Autodesk Inventor part; units mm, degrees
(part 2 of 6)
sketch "Sketch18" plane through (0, 0, 19) normal (0, 0, 1) x (1, 0, 0)
  line L0 (103.6499, -134.3094) -> (100.1144, -130.7739) projected
  line L1 (100.1144, -130.7739) -> (91.3463, -139.542) projected
  line L2 (91.3463, -139.542) -> (94.8818, -143.0776) projected
  line L3 (94.8818, -143.0776) -> (103.6499, -134.3094) projected
  line L4 (96.296, -141.6633) -> (94.8818, -145.906) projected
  line L5 (94.8818, -145.906) -> (106.4783, -134.3094) projected
  line L6 (106.4783, -134.3094) -> (102.2357, -135.7236) projected
  line L7 (102.2357, -135.7236) -> (96.296, -141.6633) projected
  line L8 (101.5286, -129.3597) -> (100.1144, -130.7739) projected
  line L9 (100.1144, -130.7739) -> (102.2357, -132.8952) projected
  line L10 (102.2357, -132.8952) -> (106.4783, -134.3094) projected
  line L11 (106.4783, -134.3094) -> (101.5286, -129.3597) projected
  line L12 (106.4783, -134.3094) -> (102.2357, -135.7236) projected
  line L13 (102.2357, -132.8952) -> (106.4783, -134.3094) projected
  line L14 (102.2357, -135.7236) -> (102.2357, -132.8952) projected
  line L15 (89.9321, -140.9562) -> (91.3463, -139.542) projected
  line L16 (89.9321, -140.9562) -> (94.8818, -145.906) projected
  line L17 (94.8818, -145.906) -> (93.4676, -141.6633) projected
  line L18 (93.4676, -141.6633) -> (91.3463, -139.542) projected
  line L19 (94.8818, -145.906) -> (93.4676, -141.6633) projected
  line L20 (96.296, -141.6633) -> (94.8818, -145.906) projected
  line L21 (93.4676, -141.6633) -> (96.296, -141.6633) projected
  line L22 (6.2, -154.1002) -> (-6.2, -154.1002) projected
  line L23 (-6.2, -154.1002) -> (-6.2, -159.1002) projected
  line L24 (-6.2, -159.1002) -> (6.2, -159.1002) projected
  line L25 (6.2, -159.1002) -> (6.2, -154.1002) projected
  line L26 (-102.2357, -132.8952) -> (-102.2357, -135.7236) projected
  line L27 (-106.4783, -134.3094) -> (-102.2357, -132.8952) projected
  line L28 (-102.2357, -135.7236) -> (-106.4783, -134.3094) projected
  line L29 (-102.2357, -135.7236) -> (-106.4783, -134.3094) projected
  line L30 (-106.4783, -134.3094) -> (-94.8818, -145.906) projected
  line L31 (-94.8818, -145.906) -> (-96.296, -141.6633) projected
  line L32 (-96.296, -141.6633) -> (-102.2357, -135.7236) projected
  line L33 (-89.9321, -140.9562) -> (-91.3463, -139.542) projected
  line L34 (-91.3463, -139.542) -> (-93.4676, -141.6633) projected
  line L35 (-93.4676, -141.6633) -> (-94.8818, -145.906) projected
  line L36 (-94.8818, -145.906) -> (-89.9321, -140.9562) projected
  line L37 (-103.6499, -134.3094) -> (-94.8818, -143.0776) projected
  line L38 (-94.8818, -143.0776) -> (-91.3463, -139.542) projected
  line L39 (-91.3463, -139.542) -> (-100.1144, -130.7739) projected
  line L40 (-100.1144, -130.7739) -> (-103.6499, -134.3094) projected
  line L41 (-101.5286, -129.3597) -> (-100.1144, -130.7739) projected
  line L42 (-101.5286, -129.3597) -> (-106.4783, -134.3094) projected
  line L43 (-106.4783, -134.3094) -> (-102.2357, -132.8952) projected
  line L44 (-102.2357, -132.8952) -> (-100.1144, -130.7739) projected
  line L45 (-89.9321, -1.6439) -> (-91.3463, -3.0581) projected
  line L46 (-89.9321, -1.6439) -> (-94.8818, 3.3058) projected
  line L47 (-94.8818, 3.3058) -> (-93.4676, -0.9368) projected
  line L48 (-93.4676, -0.9368) -> (-91.3463, -3.0581) projected
  line L49 (-96.296, -0.9368) -> (-94.8818, 3.3058) projected
  line L50 (-94.8818, 3.3058) -> (-106.4783, -8.2907) projected
  line L51 (-106.4783, -8.2907) -> (-102.2357, -6.8765) projected
  line L52 (-102.2357, -6.8765) -> (-96.296, -0.9368) projected
  line L53 (-101.5286, -13.2405) -> (-100.1144, -11.8263) projected
  line L54 (-100.1144, -11.8263) -> (-102.2357, -9.7049) projected
  line L55 (-102.2357, -9.7049) -> (-106.4783, -8.2907) projected
  line L56 (-106.4783, -8.2907) -> (-101.5286, -13.2405) projected
  line L57 (-103.6499, -8.2907) -> (-100.1144, -11.8263) projected
  line L58 (-100.1144, -11.8263) -> (-91.3463, -3.0581) projected
  line L59 (-91.3463, -3.0581) -> (-94.8818, 0.4774) projected
  line L60 (-94.8818, 0.4774) -> (-103.6499, -8.2907) projected
  line L61 (91.3463, -3.0581) -> (100.1144, -11.8263) projected
  line L62 (100.1144, -11.8263) -> (103.6499, -8.2907) projected
  line L63 (103.6499, -8.2907) -> (94.8818, 0.4774) projected
  line L64 (94.8818, 0.4774) -> (91.3463, -3.0581) projected
  line L65 (-6.2, 11.5) -> (6.2, 11.5) projected
  line L66 (6.2, 11.5) -> (6.2, 16.5) projected
  line L67 (6.2, 16.5) -> (-6.2, 16.5) projected
  line L68 (-6.2, 16.5) -> (-6.2, 11.5) projected
  point P0 (0, 0)
  point P1 (-106.4783, -8.2907)
extrude "Extrusion17" cut sketch "Sketch18" against normal blind 9
sketch "Sketch27" plane through (0, 0, 19) normal (0, 0, 1) x (1, 0, 0)
  arc A0 (0.7519, -14.6599) -> (-0.7481, -14.6599) centre (0.0019, -13.9985) ccw
  arc A1 (-0.7481, 14.663) -> (0.7519, 14.663) centre (0.0019, 14.0015) ccw
  arc A2 (-76.7327, -25.4047) -> (-77.7933, -26.4653) centre (-77.7307, -25.4673) ccw
  arc A3 (-77.723, -116.1493) -> (-76.6623, -117.21) centre (-77.6603, -117.1473) ccw
  arc A4 (-0.7284, -128.0101) -> (0.7716, -128.0101) centre (0.0216, -128.6716) ccw
  arc A5 (76.7885, -117.2378) -> (77.8491, -116.1771) centre (77.7865, -117.1752) ccw
  arc A6 (77.8163, -26.5003) -> (76.7557, -25.4397) centre (77.7537, -25.5023) ccw
  arc A7 (97.4901, -4.7053) -> (98.5507, -5.7659) centre (97.5527, -5.7033) ccw
  arc A8 (-98.5277, -5.7309) -> (-97.4671, -4.6703) centre (-97.5297, -5.6683) ccw
  arc A9 (-97.3967, -137.9444) -> (-98.4574, -136.8837) centre (-97.4593, -136.9463) ccw
  arc A10 (0.7716, -157.333) -> (-0.7284, -157.333) centre (0.0216, -156.6716) ccw
  arc A11 (98.5835, -136.9115) -> (97.5229, -137.9722) centre (97.5855, -136.9741) ccw
  point P0 (0, 0)
  constraints: 24 point on circle, 12 centre point, 48 other
hole "Hole4" at (0.0216, -128.6716, 19) at (77.7865, -117.1752, 19) at (77.7537, -25.5023, 19) at (0.0019, -13.9985, 19) at (-77.7307, -25.4673, 19) at (-77.6603, -117.1473, 19) direction (0, 0, -1) diameter 3 depth 24
sketch "Sketch28" plane through (0, 0, -5) normal (0, 0, -1) x (-1, 0, 0)
  circle A0 centre (-0.0019, -13.9985) radius 1.5 projected
  circle A1 centre (77.7307, -25.4673) radius 1.5 projected
  circle A2 centre (77.6603, -117.1473) radius 1.5 projected
  circle A3 centre (-0.0216, -128.6716) radius 1.5 projected
  circle A4 centre (-77.7865, -117.1752) radius 1.5 projected
  circle A5 centre (-77.7537, -25.5023) radius 1.5 projected
  line L0 (3.2486, -14.0007) -> (1.6214, -16.8146)
  line L1 (1.6214, -16.8146) -> (-1.6291, -16.8124)
  line L2 (-1.6291, -16.8124) -> (-3.2524, -13.9963)
  line L3 (-3.2524, -13.9963) -> (-1.6252, -11.1823)
  line L4 (-1.6252, -11.1823) -> (1.6252, -11.1846)
  line L5 (1.6252, -11.1846) -> (3.2486, -14.0007)
  line L6 (80.4442, -22.8741) -> (81.3332, -26.5207)
  line L7 (81.3332, -26.5207) -> (78.6197, -29.1139)
  line L8 (78.6197, -29.1139) -> (75.0172, -28.0605)
  line L9 (75.0172, -28.0605) -> (74.1282, -24.4139)
  line L10 (74.1282, -24.4139) -> (76.8417, -21.8207)
  line L11 (76.8417, -21.8207) -> (80.4442, -22.8741)
  line L12 (80.3739, -119.7405) -> (76.7714, -120.7939)
  line L13 (76.7714, -120.7939) -> (74.0578, -118.2007)
  line L14 (74.0578, -118.2007) -> (74.9468, -114.5542)
  line L15 (74.9468, -114.5542) -> (78.5493, -113.5008)
  line L16 (78.5493, -113.5008) -> (81.2629, -116.094)
  line L17 (81.2629, -116.094) -> (80.3739, -119.7405)
  line L18 (-0.0216, -132.2511) -> (-3.1216, -130.4614)
  line L19 (-3.1216, -130.4614) -> (-3.1216, -126.8818)
  line L20 (-3.1216, -126.8818) -> (-0.0216, -125.092)
  line L21 (-0.0216, -125.092) -> (3.0784, -126.8818)
  line L22 (3.0784, -126.8818) -> (3.0784, -130.4614)
  line L23 (3.0784, -130.4614) -> (-0.0216, -132.2511)
  line L24 (-78.6286, -113.5175) -> (-75.0399, -114.6171)
  line L25 (-75.0399, -114.6171) -> (-74.1979, -118.2748)
  line L26 (-74.1979, -118.2748) -> (-76.9445, -120.8328)
  line L27 (-76.9445, -120.8328) -> (-80.5331, -119.7332)
  line L28 (-80.5331, -119.7332) -> (-81.3752, -116.0755)
  line L29 (-81.3752, -116.0755) -> (-78.6286, -113.5175)
  line L30 (-76.9117, -21.8446) -> (-74.165, -24.4027)
  line L31 (-74.165, -24.4027) -> (-75.0071, -28.0604)
  line L32 (-75.0071, -28.0604) -> (-78.5957, -29.16)
  line L33 (-78.5957, -29.16) -> (-81.3424, -26.6019)
  line L34 (-81.3424, -26.6019) -> (-80.5003, -22.9442)
  line L35 (-80.5003, -22.9442) -> (-76.9117, -21.8446)
  circle A6 centre (77.7307, -25.4673) radius 1.5 projected
  circle A7 centre (-77.7537, -25.5023) radius 1.5 projected
  circle A8 centre (-0.0216, -128.6716) radius 1.5 projected
  circle A9 centre (-77.7865, -117.1752) radius 1.5 projected
  circle A10 centre (-0.0019, -13.9985) radius 1.5 projected
  circle A11 centre (77.6603, -117.1473) radius 1.5 projected
  circle A12 centre (0, 5.5) radius 5 projected
  circle A13 centre (-91.4877, -130.9153) radius 5 projected
  circle A14 centre (91.4877, -130.9153) radius 5 projected
  circle A15 centre (91.4877, -11.6848) radius 5 projected
  circle A16 centre (0, -148.1002) radius 5 projected
  circle A17 centre (-91.4877, -11.6848) radius 5 projected
  line L36 (-90.7904, -117.2044) -> (-78.2393, -130.6805)
  line L37 (-90.7904, -25.3958) -> (-78.2393, -11.9196)
  line L38 (90.9578, -25.2283) -> (78.2393, -11.9196)
  line L39 (78.2393, -130.6805) -> (90.9578, -117.3718)
  line L40 (-9.202, -138.2888) -> (9.202, -138.2888)
  point P0 (0, 0)
  point P1 (0, -11.1835)
  dimension "d396" = 3.2505
  dimension "d397" = 3.2505
  dimension "d398" = 3.2505
  dimension "d400" = 3.2505
  dimension "d401" = 3.2505
  dimension "d416" = 3.1
  constraints: 82 end point, 6 coincident, 5 perpendicular, 1 horizontal, 1 midpoint, 1 vertical alignment, 78 other
  measures "d396" distance of L0.start A0.centre
  measures "d397" distance from line of L6 A1.centre
  measures "d398" distance from line of L17 A2.centre
  measures "d400" distance from line of A4.centre L26
  measures "d401" distance from line of L33 A5.centre
  measures "d416" distance from line of L21 A3.centre
extrude "Extrusion27" cut sketch "Sketch28" against normal blind 2.4 contours A0 | A1 | A2 | A3 | A4 | A5 | L0 L1 L2 L3 L4 L5 | L6 L7 L8 L9 L10 L11 | L12 L13 L14 L15 L16 L17 | L18 L19 L20 L21 L22 L23 | L24 L25 L26 L27 L28 L29 | L30 L31 L32 L33 L34 L35
sketch "Sketch30" plane through (0, 0, 10) normal (0, 0, 1) x (1, 0, 0)
  line L0 (-100.1144, -130.7739) -> (-83.8509, -114.5104) projected
  line L1 (-83.8509, -114.5104) -> (-80.3154, -110.9749) projected
  line L2 (-80.3154, -110.9749) -> (-71.5473, -119.743) projected
  line L3 (-71.5473, -119.743) -> (-75.0828, -123.2786) projected
  line L4 (-75.0828, -123.2786) -> (-91.3463, -139.542) projected
  line L5 (-100.1144, -130.7739) -> (-91.3463, -139.542) projected
  line L6 (-6.2, -154.1002) -> (-6.2, -131.1002) projected
  line L7 (-6.2, -131.1002) -> (-6.2, -126.1002) projected
  line L8 (-6.2, -126.1002) -> (6.2, -126.1002) projected
  line L9 (6.2, -126.1002) -> (6.2, -131.1002) projected
  line L10 (6.2, -131.1002) -> (6.2, -154.1002) projected
  line L11 (-6.2, -154.1002) -> (6.2, -154.1002) projected
  line L12 (-91.3463, -3.0581) -> (-75.0828, -19.3216) projected
  line L13 (-75.0828, -19.3216) -> (-71.5473, -22.8571) projected
  line L14 (-71.5473, -22.8571) -> (-80.3154, -31.6252) projected
  line L15 (-80.3154, -31.6252) -> (-83.8509, -28.0897) projected
  line L16 (-83.8509, -28.0897) -> (-100.1144, -11.8263) projected
  line L17 (-91.3463, -3.0581) -> (-100.1144, -11.8263) projected
  line L18 (91.3463, -139.542) -> (75.0828, -123.2786) projected
  line L19 (75.0828, -123.2786) -> (71.5473, -119.743) projected
  line L20 (71.5473, -119.743) -> (80.3154, -110.9749) projected
  line L21 (80.3154, -110.9749) -> (83.8509, -114.5104) projected
  line L22 (83.8509, -114.5104) -> (100.1144, -130.7739) projected
  line L23 (91.3463, -139.542) -> (100.1144, -130.7739) projected
  line L24 (76.8724, -48.8001) -> (88.2822, -48.8001) projected
  line L25 (88.2822, -48.8001) -> (94.3529, -27.4901) projected
  line L26 (94.3529, -27.4901) -> (106.8333, -15.0097) projected
  arc A0 (106.8333, -15.0097) -> (88.1629, 3.6608) centre (97.4981, -5.6744) ccw projected
  line L27 (88.1629, 3.6608) -> (75.6824, -8.8196) projected
  line L28 (75.6824, -8.8196) -> (57.202, -21.3001) projected
  line L29 (57.202, -21.3001) -> (38.202, -31.3001) projected
  line L30 (38.202, -31.3001) -> (19.202, -21.3001) projected
  line L31 (19.202, -21.3001) -> (13.202, -3.65) projected
  line L32 (13.202, -3.65) -> (13.202, 14) projected
  arc A1 (13.202, 14) -> (-13.202, 14) centre (0, 14) ccw projected
  line L33 (-13.202, 14) -> (-13.202, -3.65) projected
  line L34 (-13.202, -3.65) -> (-19.202, -21.3001) projected
  line L35 (-19.202, -21.3001) -> (-38.202, -31.3001) projected
  line L36 (-38.202, -31.3001) -> (-57.202, -21.3001) projected
  line L37 (-57.202, -21.3001) -> (-75.6824, -8.8196) projected
  line L38 (-75.6824, -8.8196) -> (-88.1629, 3.6608) projected
  arc A2 (-88.1629, 3.6608) -> (-106.8333, -15.0097) centre (-97.4981, -5.6744) ccw projected
  line L39 (-106.8333, -15.0097) -> (-94.3529, -27.4901) projected
  line L40 (-94.3529, -27.4901) -> (-76.3482, -71.3001) projected
  line L41 (-76.3482, -71.3001) -> (-94.3529, -115.1101) projected
  line L42 (-94.3529, -115.1101) -> (-106.8333, -127.5905) projected
  arc A3 (-106.8333, -127.5905) -> (-88.1629, -146.2609) centre (-97.4981, -136.9257) ccw projected
  line L43 (-88.1629, -146.2609) -> (-75.6824, -133.7805) projected
  line L44 (-75.6824, -133.7805) -> (-57.202, -121.3001) projected
  line L45 (-57.202, -121.3001) -> (-38.202, -111.3001) projected
  line L46 (-38.202, -111.3001) -> (-19.202, -121.3001) projected
  line L47 (-19.202, -121.3001) -> (-13.202, -138.9501) projected
  line L48 (-13.202, -138.9501) -> (-13.202, -156.6002) projected
  arc A4 (-13.202, -156.6002) -> (13.202, -156.6002) centre (0, -156.6002) ccw projected
  line L49 (13.202, -156.6002) -> (13.202, -138.9501) projected
  line L50 (13.202, -138.9501) -> (19.202, -121.3001) projected
  line L51 (19.202, -121.3001) -> (38.202, -111.3001) projected
  line L52 (38.202, -111.3001) -> (57.202, -121.3001) projected
  line L53 (57.202, -121.3001) -> (75.6824, -133.7805) projected
  line L54 (75.6824, -133.7805) -> (88.1629, -146.2609) projected
  arc A5 (88.1629, -146.2609) -> (106.8333, -127.5905) centre (97.4981, -136.9257) ccw projected
  line L55 (106.8333, -127.5905) -> (94.3529, -115.1101) projected
  line L56 (94.3529, -115.1101) -> (88.2822, -93.8001) projected
  line L57 (88.2822, -93.8001) -> (76.8724, -93.8001) projected
  line L58 (76.8724, -93.8001) -> (76.8724, -48.8001) projected
  line L59 (6.2, -16.5) -> (-6.2, -16.5) projected
  line L60 (-6.2, -16.5) -> (-6.2, -11.5) projected
  line L61 (-6.2, -11.5) -> (-6.2, 11.5) projected
  line L62 (6.2, 11.5) -> (-6.2, 11.5) projected
  line L63 (6.2, 11.5) -> (6.2, -11.5) projected
  line L64 (6.2, -11.5) -> (6.2, -16.5) projected
  line L65 (100.1144, -11.8263) -> (83.8509, -28.0897) projected
  line L66 (83.8509, -28.0897) -> (80.3154, -31.6252) projected
  line L67 (80.3154, -31.6252) -> (71.5473, -22.8571) projected
  line L68 (71.5473, -22.8571) -> (75.0828, -19.3216) projected
  line L69 (75.0828, -19.3216) -> (91.3463, -3.0581) projected
  line L70 (100.1144, -11.8263) -> (91.3463, -3.0581) projected
  line L71 (-6.2, 11.5) -> (6.2, 11.5)
  line L72 (6.2, 11.5) -> (6.2, 17.5)
  line L73 (6.2, 17.5) -> (-6.2, 17.5)
  line L74 (-6.2, 17.5) -> (-6.2, 11.5)
  line L75 (0, 11.5) -> (0, 17.5)
  line L76 (0, 17.5) -> (4.5, 17.5)
  line L77 (4.5, 17.5) -> (4.5, 11.5)
  line L78 (4.5, 11.5) -> (0, 11.5)
  line L79 (0, 11.5) -> (-4.5, 11.5)
  line L80 (-4.5, 11.5) -> (-4.5, 17.5)
  line L81 (-4.5, 17.5) -> (0, 17.5)
  line L82 (0, 17.5) -> (0, 11.5)
  line L83 (-100.1144, -11.8263) -> (-91.3463, -3.0581)
  line L84 (-91.3463, -3.0581) -> (-95.5889, 1.1845)
  line L85 (-95.5889, 1.1845) -> (-104.357, -7.5836)
  line L86 (-104.357, -7.5836) -> (-100.1144, -11.8263)
  line L87 (-95.7303, -7.4422) -> (-92.5483, -4.2602)
  line L88 (-92.5483, -4.2602) -> (-96.791, -0.0176)
  line L89 (-96.791, -0.0176) -> (-99.973, -3.1996)
  line L90 (-99.973, -3.1996) -> (-95.7303, -7.4422)
  line L91 (-95.7303, -7.4422) -> (-98.9123, -10.6242)
  line L92 (-98.9123, -10.6242) -> (-103.1549, -6.3815)
  line L93 (-103.1549, -6.3815) -> (-99.973, -3.1996)
  line L94 (-99.973, -3.1996) -> (-95.7303, -7.4422)
  line L95 (-100.1144, -130.7739) -> (-91.3463, -139.542)
  line L96 (-91.3463, -139.542) -> (-95.5889, -143.7847)
  line L97 (-95.5889, -143.7847) -> (-104.357, -135.0165)
  line L98 (-104.357, -135.0165) -> (-100.1144, -130.7739)
  line L99 (-95.7303, -135.158) -> (-98.9123, -131.976)
  line L100 (-98.9123, -131.976) -> (-103.1549, -136.2186)
  line L101 (-103.1549, -136.2186) -> (-99.973, -139.4006)
  line L102 (-99.973, -139.4006) -> (-95.7303, -135.158)
  line L103 (-95.7303, -135.158) -> (-99.973, -139.4006)
  line L104 (-99.973, -139.4006) -> (-96.791, -142.5826)
  line L105 (-96.791, -142.5826) -> (-92.5483, -138.3399)
  line L106 (-92.5483, -138.3399) -> (-95.7303, -135.158)
  line L107 (-6.2, -154.1002) -> (6.2, -154.1002)
  line L108 (6.2, -154.1002) -> (6.2, -160.1002)
  line L109 (6.2, -160.1002) -> (-6.2, -160.1002)
  line L110 (-6.2, -160.1002) -> (-6.2, -154.1002)
  line L111 (0, -154.1002) -> (0, -160.1002)
  line L112 (0, -160.1002) -> (-4.5, -160.1002)
  line L113 (-4.5, -160.1002) -> (-4.5, -154.1002)
  line L114 (-4.5, -154.1002) -> (0, -154.1002)
  line L115 (0, -154.1002) -> (0, -160.1002)
  line L116 (0, -160.1002) -> (4.5, -160.1002)
  line L117 (4.5, -160.1002) -> (4.5, -154.1002)
  line L118 (4.5, -154.1002) -> (0, -154.1002)
  line L119 (91.3463, -139.542) -> (100.1144, -130.7739)
  line L120 (100.1144, -130.7739) -> (104.357, -135.0165)
  line L121 (104.357, -135.0165) -> (95.5889, -143.7847)
  line L122 (95.5889, -143.7847) -> (91.3463, -139.542)
  line L123 (95.7303, -135.158) -> (99.973, -139.4006)
  line L124 (99.973, -139.4006) -> (96.791, -142.5826)
  line L125 (96.791, -142.5826) -> (92.5483, -138.3399)
  line L126 (92.5483, -138.3399) -> (95.7303, -135.158)
  line L127 (95.7303, -135.158) -> (99.973, -139.4006)
  line L128 (99.973, -139.4006) -> (103.1549, -136.2186)
  line L129 (103.1549, -136.2186) -> (98.9123, -131.976)
  line L130 (98.9123, -131.976) -> (95.7303, -135.158)
  line L131 (91.3463, -3.0581) -> (100.1144, -11.8263)
  line L132 (100.1144, -11.8263) -> (104.357, -7.5836)
  line L133 (104.357, -7.5836) -> (95.5889, 1.1845)
  line L134 (95.5889, 1.1845) -> (91.3463, -3.0581)
  line L135 (95.7303, -7.4422) -> (99.973, -3.1996)
  line L136 (99.973, -3.1996) -> (96.791, -0.0176)
  line L137 (96.791, -0.0176) -> (92.5483, -4.2602)
  line L138 (92.5483, -4.2602) -> (95.7303, -7.4422)
  line L139 (95.7303, -7.4422) -> (98.9123, -10.6242)
  line L140 (98.9123, -10.6242) -> (103.1549, -6.3815)
  line L141 (103.1549, -6.3815) -> (99.973, -3.1996)
  line L142 (99.973, -3.1996) -> (95.7303, -7.4422)
  point P0 (0, 0)
  point P1 (96.791, -0.0176)
  point P2 (-96.791, -142.5826)
  point P3 (-103.1549, -136.2186)
  point P4 (-96.791, -0.0176)
  point P5 (-103.1549, -6.3815)
  point P6 (4.5, 17.5)
  dimension "d455" = 6
  dimension "d456" = 4.5
  dimension "d457" = 4.5
  dimension "d458" = 1.7
  dimension "d459" = 12.4
  dimension "d460" = 6
  dimension "d461" = 4.5
  dimension "d462" = 4.5
  dimension "d463" = 6
  dimension "d464" = 4.5
  dimension "d465" = 4.5
  dimension "d466" = 6
  dimension "d467" = 4.5
  dimension "d468" = 4.5
  dimension "d472" = 6
  dimension "d473" = 4.5
  dimension "d474" = 4.5
  dimension "d475" = 4.5
  dimension "d476" = 4.5
  dimension "d477" = 6
  dimension "d478" = 154.5851
  dimension "d479" = 147.5831
  dimension "d480" = 147.5831
  constraints: 144 end point, 39 equal length, 24 perpendicular, 10 midpoint, 7 point on line
  measures "d455" distance of L72.end L62.start
  measures "d456" distance of L75.end L76.end
  measures "d457" distance of L75.start L79.end
  measures "d458" distance between parallel lines of L80 L74
  measures "d459" distance of L72.end L73.end
  measures "d460" distance of L84.end L12.start
  measures "d461" distance between parallel lines of L88 L90
  measures "d462" distance between parallel lines of L90 L92
  measures "d463" distance of L4.end L96.end
  measures "d464" distance between parallel lines of L100 L102
  measures "d465" distance between parallel lines of L102 L105
  measures "d466" distance of L10.end L108.end
  measures "d467" distance between parallel lines of L113 L111
  measures "d468" distance between parallel lines of L111 L117
  measures "d472" distance of L18.start L121.end
  measures "d473" distance between parallel lines of L125 L123
  measures "d474" distance between parallel lines of L129 L123
  measures "d475" distance between parallel lines of L137 L135
  measures "d476" distance between parallel lines of L135 L140
  measures "d477" distance of L133.end L69.end
  measures "d478" distance between parallel lines of L55 L101
  measures "d479" distance between parallel lines of L65 L89
  measures "d480" distance between parallel lines of L65 L93
extrude "Extrusion29" add sketch "Sketch30" along normal blind 9 contours L5 L100 L97 L98 | L5 L96 L97 L105 | L11 L113 L109 L110 | L11 L108 L109 L117 | L17 L88 L85 L84 | L17 L86 L85 L92 | L23 L125 L121 L122 | L23 L120 L121 L129 | L62 L77 L73 L72 | L74 L73 L80 L62 | L70 L140 L133 L132 | L70 L134 L133 L137
sketch "Sketch31" plane through (0, 0, 10) normal (0, 0, 1) x (1, 0, 0)
  line L0 (76.8724, -48.8001) -> (88.2822, -48.8001) projected
  line L1 (88.2822, -48.8001) -> (94.3529, -27.4901) projected
  line L2 (94.3529, -27.4901) -> (106.8333, -15.0097) projected
  arc A0 (106.8333, -15.0097) -> (88.1629, 3.6608) centre (97.4981, -5.6744) ccw projected
  line L3 (88.1629, 3.6608) -> (75.6824, -8.8196) projected
  line L4 (75.6824, -8.8196) -> (57.202, -21.3001) projected
  line L5 (57.202, -21.3001) -> (38.202, -31.3001) projected
  line L6 (38.202, -31.3001) -> (19.202, -21.3001) projected
  line L7 (19.202, -21.3001) -> (13.202, -3.65) projected
  line L8 (13.202, -3.65) -> (13.202, 14) projected
  arc A1 (13.202, 14) -> (-13.202, 14) centre (0, 14) ccw projected
  line L9 (-13.202, 14) -> (-13.202, -3.65) projected
  line L10 (-13.202, -3.65) -> (-19.202, -21.3001) projected
  line L11 (-19.202, -21.3001) -> (-38.202, -31.3001) projected
  line L12 (-38.202, -31.3001) -> (-57.202, -21.3001) projected
  line L13 (-57.202, -21.3001) -> (-75.6824, -8.8196) projected
  line L14 (-75.6824, -8.8196) -> (-88.1629, 3.6608) projected
  arc A2 (-88.1629, 3.6608) -> (-106.8333, -15.0097) centre (-97.4981, -5.6744) ccw projected
  line L15 (-106.8333, -15.0097) -> (-94.3529, -27.4901) projected
  line L16 (-94.3529, -27.4901) -> (-76.3482, -71.3001) projected
  line L17 (-76.3482, -71.3001) -> (-94.3529, -115.1101) projected
  line L18 (-94.3529, -115.1101) -> (-106.8333, -127.5905) projected
  arc A3 (-106.8333, -127.5905) -> (-88.1629, -146.2609) centre (-97.4981, -136.9257) ccw projected
  line L19 (-88.1629, -146.2609) -> (-75.6824, -133.7805) projected
  line L20 (-75.6824, -133.7805) -> (-57.202, -121.3001) projected
  line L21 (-57.202, -121.3001) -> (-38.202, -111.3001) projected
  line L22 (-38.202, -111.3001) -> (-19.202, -121.3001) projected
  line L23 (-19.202, -121.3001) -> (-13.202, -138.9501) projected
  line L24 (-13.202, -138.9501) -> (-13.202, -156.6002) projected
  arc A4 (-13.202, -156.6002) -> (13.202, -156.6002) centre (0, -156.6002) ccw projected
  line L25 (13.202, -156.6002) -> (13.202, -138.9501) projected
  line L26 (13.202, -138.9501) -> (19.202, -121.3001) projected
  line L27 (19.202, -121.3001) -> (38.202, -111.3001) projected
  line L28 (38.202, -111.3001) -> (57.202, -121.3001) projected
  line L29 (57.202, -121.3001) -> (75.6824, -133.7805) projected
  line L30 (75.6824, -133.7805) -> (88.1629, -146.2609) projected
  arc A5 (88.1629, -146.2609) -> (106.8333, -127.5905) centre (97.4981, -136.9257) ccw projected
  line L31 (106.8333, -127.5905) -> (94.3529, -115.1101) projected
  line L32 (94.3529, -115.1101) -> (88.2822, -93.8001) projected
  line L33 (88.2822, -93.8001) -> (76.8724, -93.8001) projected
  line L34 (76.8724, -93.8001) -> (76.8724, -48.8001) projected
  line L35 (-91.3463, -139.542) -> (-95.5889, -143.7847) projected
  line L36 (-95.5889, -143.7847) -> (-96.791, -142.5826) projected
  line L37 (-96.791, -142.5826) -> (-92.5483, -138.3399) projected
  line L38 (-98.9123, -131.976) -> (-92.5483, -138.3399) projected
  line L39 (-98.9123, -131.976) -> (-103.1549, -136.2186) projected
  line L40 (-103.1549, -136.2186) -> (-104.357, -135.0165) projected
  line L41 (-104.357, -135.0165) -> (-100.1144, -130.7739) projected
  line L42 (-100.1144, -130.7739) -> (-83.8509, -114.5104) projected
  line L43 (-83.8509, -114.5104) -> (-80.3154, -110.9749) projected
  line L44 (-80.3154, -110.9749) -> (-71.5473, -119.743) projected
  line L45 (-71.5473, -119.743) -> (-75.0828, -123.2786) projected
  line L46 (-75.0828, -123.2786) -> (-91.3463, -139.542) projected
  line L47 (100.1144, -130.7739) -> (104.357, -135.0165) projected
  line L48 (104.357, -135.0165) -> (103.1549, -136.2186) projected
  line L49 (103.1549, -136.2186) -> (98.9123, -131.976) projected
  line L50 (92.5483, -138.3399) -> (98.9123, -131.976) projected
  line L51 (92.5483, -138.3399) -> (96.791, -142.5826) projected
  line L52 (96.791, -142.5826) -> (95.5889, -143.7847) projected
  line L53 (95.5889, -143.7847) -> (91.3463, -139.542) projected
  line L54 (91.3463, -139.542) -> (75.0828, -123.2786) projected
  line L55 (75.0828, -123.2786) -> (71.5473, -119.743) projected
  line L56 (71.5473, -119.743) -> (80.3154, -110.9749) projected
  line L57 (80.3154, -110.9749) -> (83.8509, -114.5104) projected
  line L58 (83.8509, -114.5104) -> (100.1144, -130.7739) projected
  line L59 (-100.1144, -11.8263) -> (-104.357, -7.5836) projected
  line L60 (-104.357, -7.5836) -> (-103.1549, -6.3815) projected
  line L61 (-103.1549, -6.3815) -> (-98.9123, -10.6242) projected
  line L62 (-92.5483, -4.2602) -> (-98.9123, -10.6242) projected
  line L63 (-92.5483, -4.2602) -> (-96.791, -0.0176) projected
  line L64 (-96.791, -0.0176) -> (-95.5889, 1.1845) projected
  line L65 (-95.5889, 1.1845) -> (-91.3463, -3.0581) projected
  line L66 (-91.3463, -3.0581) -> (-75.0828, -19.3216) projected
  line L67 (-75.0828, -19.3216) -> (-71.5473, -22.8571) projected
  line L68 (-71.5473, -22.8571) -> (-80.3154, -31.6252) projected
  line L69 (-80.3154, -31.6252) -> (-83.8509, -28.0897) projected
  line L70 (-83.8509, -28.0897) -> (-100.1144, -11.8263) projected
  line L71 (6.2, 17.5) -> (6.2, 11.5) projected
  line L72 (6.2, 11.5) -> (6.2, -11.5) projected
  line L73 (6.2, -11.5) -> (6.2, -16.5) projected
  line L74 (6.2, -16.5) -> (-6.2, -16.5) projected
  line L75 (-6.2, -16.5) -> (-6.2, -11.5) projected
  line L76 (-6.2, -11.5) -> (-6.2, 11.5) projected
  line L77 (-6.2, 11.5) -> (-6.2, 17.5) projected
  line L78 (-6.2, 17.5) -> (-4.5, 17.5) projected
  line L79 (-4.5, 17.5) -> (-4.5, 11.5) projected
  line L80 (4.5, 11.5) -> (-4.5, 11.5) projected
  line L81 (4.5, 11.5) -> (4.5, 17.5) projected
  line L82 (4.5, 17.5) -> (6.2, 17.5) projected
  line L83 (104.357, -7.5836) -> (100.1144, -11.8263) projected
  line L84 (100.1144, -11.8263) -> (83.8509, -28.0897) projected
  line L85 (83.8509, -28.0897) -> (80.3154, -31.6252) projected
  line L86 (80.3154, -31.6252) -> (71.5473, -22.8571) projected
  line L87 (71.5473, -22.8571) -> (75.0828, -19.3216) projected
  line L88 (75.0828, -19.3216) -> (91.3463, -3.0581) projected
  line L89 (91.3463, -3.0581) -> (95.5889, 1.1845) projected
  line L90 (95.5889, 1.1845) -> (96.791, -0.0176) projected
  line L91 (96.791, -0.0176) -> (92.5483, -4.2602) projected
  line L92 (98.9123, -10.6242) -> (92.5483, -4.2602) projected
  line L93 (98.9123, -10.6242) -> (103.1549, -6.3815) projected
  line L94 (103.1549, -6.3815) -> (104.357, -7.5836) projected
  line L95 (-6.2, -160.1002) -> (-6.2, -154.1002) projected
  line L96 (-6.2, -154.1002) -> (-6.2, -131.1002) projected
  line L97 (-6.2, -131.1002) -> (-6.2, -126.1002) projected
  line L98 (-6.2, -126.1002) -> (6.2, -126.1002) projected
  line L99 (6.2, -126.1002) -> (6.2, -131.1002) projected
  line L100 (6.2, -131.1002) -> (6.2, -154.1002) projected
  line L101 (6.2, -154.1002) -> (6.2, -160.1002) projected
  line L102 (6.2, -160.1002) -> (4.5, -160.1002) projected
  line L103 (4.5, -160.1002) -> (4.5, -154.1002) projected
  line L104 (-4.5, -154.1002) -> (4.5, -154.1002) projected
  line L105 (-4.5, -154.1002) -> (-4.5, -160.1002) projected
  line L106 (-4.5, -160.1002) -> (-6.2, -160.1002) projected
  line L107 (-4.5, 11.5) -> (-4.5, 17.5)
  line L108 (-4.5, 17.5) -> (4.5, 17.5)
  line L109 (4.5, 17.5) -> (4.5, 11.5)
  line L110 (4.5, 11.5) -> (-4.5, 11.5)
  line L111 (-98.9123, -10.6242) -> (-92.5483, -4.2602)
  line L112 (-92.5483, -4.2602) -> (-96.791, -0.0176)
  line L113 (-96.791, -0.0176) -> (-103.1549, -6.3815)
  line L114 (-103.1549, -6.3815) -> (-98.9123, -10.6242)
  line L115 (-98.9123, -131.976) -> (-92.5483, -138.3399)
  line L116 (-92.5483, -138.3399) -> (-96.791, -142.5826)
  line L117 (-96.791, -142.5826) -> (-103.1549, -136.2186)
  line L118 (-103.1549, -136.2186) -> (-98.9123, -131.976)
  line L119 (-4.5, -154.1002) -> (4.5, -154.1002)
  line L120 (4.5, -154.1002) -> (4.5, -160.1002)
  line L121 (4.5, -160.1002) -> (-4.5, -160.1002)
  line L122 (-4.5, -160.1002) -> (-4.5, -154.1002)
  line L123 (92.5483, -138.3399) -> (98.9123, -131.976)
  line L124 (98.9123, -131.976) -> (103.1549, -136.2186)
  line L125 (103.1549, -136.2186) -> (96.791, -142.5826)
  line L126 (96.791, -142.5826) -> (92.5483, -138.3399)
  line L127 (98.9123, -10.6242) -> (103.1549, -6.3815)
  line L128 (103.1549, -6.3815) -> (96.791, -0.0176)
  line L129 (96.791, -0.0176) -> (92.5483, -4.2602)
  line L130 (92.5483, -4.2602) -> (98.9123, -10.6242)
  point P0 (0, 0)
  dimension "d483" = 154.5851
  dimension "d484" = 90.1087
  dimension "d485" = 10.7
  dimension "d486" = 147.5831
  dimension "d487" = 66.3001
  dimension "d488" = 72.3725
  constraints: 48 end point, 15 equal length, 9 perpendicular
  measures "d483" distance between parallel lines of L31 L117
  measures "d484" distance between parallel lines of L83 L125
  measures "d485" distance between parallel lines of L83 L129
  measures "d486" distance between parallel lines of L83 L113
  measures "d487" distance between parallel lines of L33 L121
  measures "d488" distance between parallel lines of L34 L109
extrude "Extrusion30" cut sketch "Sketch31" against normal blind 10 contours L117 L39 L38 L37 | L125 L51 L50 L49 | L113 L63 L62 L61 | L81 L80 L79 L108 | L93 L92 L91 L128 | L105 L104 L103 L121
sketch "Sketch32" plane through (0, 0, 19) normal (0, 0, 1) x (1, 0, 0)
  line L0 (4.5, 17.5) -> (4.5, 11.5) projected
  line L1 (4.5, 11.5) -> (6.2, 11.5) projected
  line L2 (6.2, 11.5) -> (6.2, 17.5) projected
  line L3 (6.2, 17.5) -> (4.5, 17.5) projected
  line L4 (-4.5, 17.5) -> (-6.2, 17.5) projected
  line L5 (-6.2, 17.5) -> (-6.2, 11.5) projected
  line L6 (-6.2, 11.5) -> (-4.5, 11.5) projected
  line L7 (-4.5, 11.5) -> (-4.5, 17.5) projected
  line L8 (-103.1549, -6.3815) -> (-104.357, -7.5836) projected
  line L9 (-104.357, -7.5836) -> (-100.1144, -11.8263) projected
  line L10 (-100.1144, -11.8263) -> (-98.9123, -10.6242) projected
  line L11 (-98.9123, -10.6242) -> (-103.1549, -6.3815) projected
  line L12 (-96.791, -0.0176) -> (-92.5483, -4.2602) projected
  line L13 (-92.5483, -4.2602) -> (-91.3463, -3.0581) projected
  line L14 (-91.3463, -3.0581) -> (-95.5889, 1.1845) projected
  line L15 (-95.5889, 1.1845) -> (-96.791, -0.0176) projected
  line L16 (-92.5483, -138.3399) -> (-96.791, -142.5826) projected
  line L17 (-96.791, -142.5826) -> (-95.5889, -143.7847) projected
  line L18 (-95.5889, -143.7847) -> (-91.3463, -139.542) projected
  line L19 (-91.3463, -139.542) -> (-92.5483, -138.3399) projected
  line L20 (-98.9123, -131.976) -> (-100.1144, -130.7739) projected
  line L21 (-100.1144, -130.7739) -> (-104.357, -135.0165) projected
  line L22 (-104.357, -135.0165) -> (-103.1549, -136.2186) projected
  line L23 (-103.1549, -136.2186) -> (-98.9123, -131.976) projected
  line L24 (-4.5, -154.1002) -> (-6.2, -154.1002) projected
  line L25 (-6.2, -154.1002) -> (-6.2, -160.1002) projected
  line L26 (-6.2, -160.1002) -> (-4.5, -160.1002) projected
  line L27 (-4.5, -160.1002) -> (-4.5, -154.1002) projected
  line L28 (4.5, -154.1002) -> (4.5, -160.1002) projected
  line L29 (4.5, -160.1002) -> (6.2, -160.1002) projected
  line L30 (6.2, -160.1002) -> (6.2, -154.1002) projected
  line L31 (6.2, -154.1002) -> (4.5, -154.1002) projected
  line L32 (92.5483, -138.3399) -> (91.3463, -139.542) projected
  line L33 (91.3463, -139.542) -> (95.5889, -143.7847) projected
  line L34 (95.5889, -143.7847) -> (96.791, -142.5826) projected
  line L35 (96.791, -142.5826) -> (92.5483, -138.3399) projected
  line L36 (98.9123, -131.976) -> (103.1549, -136.2186) projected
  line L37 (103.1549, -136.2186) -> (104.357, -135.0165) projected
  line L38 (104.357, -135.0165) -> (100.1144, -130.7739) projected
  line L39 (100.1144, -130.7739) -> (98.9123, -131.976) projected
  line L40 (98.9123, -10.6242) -> (100.1144, -11.8263) projected
  line L41 (100.1144, -11.8263) -> (104.357, -7.5836) projected
  line L42 (104.357, -7.5836) -> (103.1549, -6.3815) projected
  line L43 (103.1549, -6.3815) -> (98.9123, -10.6242) projected
  line L44 (92.5483, -4.2602) -> (96.791, -0.0176) projected
  line L45 (96.791, -0.0176) -> (95.5889, 1.1845) projected
  line L46 (95.5889, 1.1845) -> (91.3463, -3.0581) projected
  line L47 (91.3463, -3.0581) -> (92.5483, -4.2602) projected
  line L48 (-4.5, 17.5) -> (-4.5, 11.5)
  line L49 (-4.5, 11.5) -> (4.5, 11.5)
  line L50 (4.5, 11.5) -> (4.5, 17.5)
  line L51 (4.5, 17.5) -> (-4.5, 17.5)
  line L52 (-96.791, -0.0176) -> (-103.1549, -6.3815)
  line L53 (-103.1549, -6.3815) -> (-98.9123, -10.6242)
  line L54 (-98.9123, -10.6242) -> (-92.5483, -4.2602)
  line L55 (-92.5483, -4.2602) -> (-96.791, -0.0176)
  line L56 (-103.1549, -136.2186) -> (-96.791, -142.5826)
  line L57 (-96.791, -142.5826) -> (-92.5483, -138.3399)
  line L58 (-92.5483, -138.3399) -> (-98.9123, -131.976)
  line L59 (-98.9123, -131.976) -> (-103.1549, -136.2186)
  line L60 (-4.5, -160.1002) -> (4.5, -160.1002)
  line L61 (4.5, -160.1002) -> (4.5, -154.1002)
  line L62 (4.5, -154.1002) -> (-4.5, -154.1002)
  line L63 (-4.5, -154.1002) -> (-4.5, -160.1002)
  line L64 (98.9123, -131.976) -> (92.5483, -138.3399)
  line L65 (92.5483, -138.3399) -> (96.791, -142.5826)
  line L66 (96.791, -142.5826) -> (103.1549, -136.2186)
  line L67 (103.1549, -136.2186) -> (98.9123, -131.976)
  line L68 (92.5483, -4.2602) -> (98.9123, -10.6242)
  line L69 (98.9123, -10.6242) -> (103.1549, -6.3815)
  line L70 (103.1549, -6.3815) -> (96.791, -0.0176)
  line L71 (96.791, -0.0176) -> (92.5483, -4.2602)
  point P0 (0, 0)
  point P1 (96.791, -0.0176)
  dimension "d491" = 0
  dimension "d492" = 231.6918
  dimension "d493" = 91.8087
  dimension "d494" = 139.8831
  dimension "d495" = 171.6002
  dimension "d496" = 1.7
  constraints: 48 end point, 13 parallel, 10 perpendicular, 1 vertical
  measures "d491" distance between parallel lines of L42 L70
  measures "d492" distance between parallel lines of L42 L58
  measures "d493" distance between parallel lines of L43 L66
  measures "d494" distance between parallel lines of L43 L54
  measures "d495" distance between parallel lines of L3 L62
  measures "d496" distance between parallel lines of L2 L50
extrude "Extrusion31" add sketch "Sketch32" against normal blind 5 contours L0 L49 L7 L51 | L52 L12 L54 L11 | L16 L56 L23 L58 | L62 L28 L60 L27 | L64 L36 L66 L35 | L68 L44 L70 L43
sketch "Sketch35" plane through (0, 0, 10) normal (0, 0, 1) x (1, 0, 0)
  line L0 (-103.1549, -6.3815) -> (-96.791, -0.0176) projected
  line L1 (-96.791, -0.0176) -> (-95.5889, 1.1845) projected
  line L2 (-95.5889, 1.1845) -> (-91.3463, -3.0581) projected
  line L3 (-91.3463, -3.0581) -> (-75.0828, -19.3216) projected
  line L4 (-75.0828, -19.3216) -> (-71.5473, -22.8571) projected
  line L5 (-71.5473, -22.8571) -> (-80.3154, -31.6252) projected
  line L6 (-80.3154, -31.6252) -> (-83.8509, -28.0897) projected
  line L7 (-83.8509, -28.0897) -> (-100.1144, -11.8263) projected
  line L8 (-100.1144, -11.8263) -> (-104.357, -7.5836) projected
  line L9 (-104.357, -7.5836) -> (-103.1549, -6.3815) projected
  line L10 (4.5, -160.1002) -> (-4.5, -160.1002) projected
  line L11 (-4.5, -160.1002) -> (-6.2, -160.1002) projected
  line L12 (-6.2, -160.1002) -> (-6.2, -154.1002) projected
  line L13 (-6.2, -154.1002) -> (-6.2, -131.1002) projected
  line L14 (-6.2, -131.1002) -> (-6.2, -126.1002) projected
  line L15 (-6.2, -126.1002) -> (6.2, -126.1002) projected
  line L16 (6.2, -126.1002) -> (6.2, -131.1002) projected
  line L17 (6.2, -131.1002) -> (6.2, -154.1002) projected
  line L18 (6.2, -154.1002) -> (6.2, -160.1002) projected
  line L19 (6.2, -160.1002) -> (4.5, -160.1002) projected
  line L20 (96.791, -0.0176) -> (103.1549, -6.3815) projected
  line L21 (103.1549, -6.3815) -> (104.357, -7.5836) projected
  line L22 (104.357, -7.5836) -> (100.1144, -11.8263) projected
  line L23 (100.1144, -11.8263) -> (83.8509, -28.0897) projected
  line L24 (83.8509, -28.0897) -> (80.3154, -31.6252) projected
  line L25 (80.3154, -31.6252) -> (71.5473, -22.8571) projected
  line L26 (71.5473, -22.8571) -> (75.0828, -19.3216) projected
  line L27 (75.0828, -19.3216) -> (91.3463, -3.0581) projected
  line L28 (91.3463, -3.0581) -> (95.5889, 1.1845) projected
  line L29 (95.5889, 1.1845) -> (96.791, -0.0176) projected
  line L30 (76.8724, -48.8001) -> (88.2822, -48.8001) projected
  line L31 (88.2822, -48.8001) -> (94.3529, -27.4901) projected
  line L32 (94.3529, -27.4901) -> (106.8333, -15.0097) projected
  arc A0 (106.8333, -15.0097) -> (88.1629, 3.6608) centre (97.4981, -5.6744) ccw projected
  line L33 (88.1629, 3.6608) -> (75.6824, -8.8196) projected
  line L34 (75.6824, -8.8196) -> (57.202, -21.3001) projected
  line L35 (57.202, -21.3001) -> (38.202, -31.3001) projected
  line L36 (38.202, -31.3001) -> (19.202, -21.3001) projected
  line L37 (19.202, -21.3001) -> (13.202, -3.65) projected
  line L38 (13.202, -3.65) -> (13.202, 14) projected
  arc A1 (13.202, 14) -> (-13.202, 14) centre (0, 14) ccw projected
  line L39 (-13.202, 14) -> (-13.202, -3.65) projected
  line L40 (-13.202, -3.65) -> (-19.202, -21.3001) projected
  line L41 (-19.202, -21.3001) -> (-38.202, -31.3001) projected
  line L42 (-38.202, -31.3001) -> (-57.202, -21.3001) projected
  line L43 (-57.202, -21.3001) -> (-75.6824, -8.8196) projected
  line L44 (-75.6824, -8.8196) -> (-88.1629, 3.6608) projected
  arc A2 (-88.1629, 3.6608) -> (-106.8333, -15.0097) centre (-97.4981, -5.6744) ccw projected
  line L45 (-106.8333, -15.0097) -> (-94.3529, -27.4901) projected
  line L46 (-94.3529, -27.4901) -> (-76.3482, -71.3001) projected
  line L47 (-76.3482, -71.3001) -> (-94.3529, -115.1101) projected
  line L48 (-94.3529, -115.1101) -> (-106.8333, -127.5905) projected
  arc A3 (-106.8333, -127.5905) -> (-88.1629, -146.2609) centre (-97.4981, -136.9257) ccw projected
  line L49 (-88.1629, -146.2609) -> (-75.6824, -133.7805) projected
  line L50 (-75.6824, -133.7805) -> (-57.202, -121.3001) projected
  line L51 (-57.202, -121.3001) -> (-38.202, -111.3001) projected
  line L52 (-38.202, -111.3001) -> (-19.202, -121.3001) projected
  line L53 (-19.202, -121.3001) -> (-13.202, -138.9501) projected
  line L54 (-13.202, -138.9501) -> (-13.202, -156.6002) projected
  arc A4 (-13.202, -156.6002) -> (13.202, -156.6002) centre (0, -156.6002) ccw projected
  line L55 (13.202, -156.6002) -> (13.202, -138.9501) projected
  line L56 (13.202, -138.9501) -> (19.202, -121.3001) projected
  line L57 (19.202, -121.3001) -> (38.202, -111.3001) projected
  line L58 (38.202, -111.3001) -> (57.202, -121.3001) projected
  line L59 (57.202, -121.3001) -> (75.6824, -133.7805) projected
  line L60 (75.6824, -133.7805) -> (88.1629, -146.2609) projected
  arc A5 (88.1629, -146.2609) -> (106.8333, -127.5905) centre (97.4981, -136.9257) ccw projected
  line L61 (106.8333, -127.5905) -> (94.3529, -115.1101) projected
  line L62 (94.3529, -115.1101) -> (88.2822, -93.8001) projected
  line L63 (88.2822, -93.8001) -> (76.8724, -93.8001) projected
  line L64 (76.8724, -93.8001) -> (76.8724, -48.8001) projected
  line L65 (-96.791, -142.5826) -> (-103.1549, -136.2186) projected
  line L66 (-103.1549, -136.2186) -> (-104.357, -135.0165) projected
  line L67 (-104.357, -135.0165) -> (-100.1144, -130.7739) projected
  line L68 (-100.1144, -130.7739) -> (-83.8509, -114.5104) projected
  line L69 (-83.8509, -114.5104) -> (-80.3154, -110.9749) projected
  line L70 (-80.3154, -110.9749) -> (-71.5473, -119.743) projected
  line L71 (-71.5473, -119.743) -> (-75.0828, -123.2786) projected
  line L72 (-75.0828, -123.2786) -> (-91.3463, -139.542) projected
  line L73 (-91.3463, -139.542) -> (-95.5889, -143.7847) projected
  line L74 (-95.5889, -143.7847) -> (-96.791, -142.5826) projected
  line L75 (103.1549, -136.2186) -> (96.791, -142.5826) projected
  line L76 (96.791, -142.5826) -> (95.5889, -143.7847) projected
  line L77 (95.5889, -143.7847) -> (91.3463, -139.542) projected
  line L78 (91.3463, -139.542) -> (75.0828, -123.2786) projected
  line L79 (75.0828, -123.2786) -> (71.5473, -119.743) projected
  line L80 (71.5473, -119.743) -> (80.3154, -110.9749) projected
  line L81 (80.3154, -110.9749) -> (83.8509, -114.5104) projected
  line L82 (83.8509, -114.5104) -> (100.1144, -130.7739) projected
  line L83 (100.1144, -130.7739) -> (104.357, -135.0165) projected
  line L84 (104.357, -135.0165) -> (103.1549, -136.2186) projected
  line L85 (-4.5, 17.5) -> (4.5, 17.5) projected
  line L86 (4.5, 17.5) -> (6.2, 17.5) projected
  line L87 (6.2, 17.5) -> (6.2, 11.5) projected
  line L88 (6.2, 11.5) -> (6.2, -11.5) projected
  line L89 (6.2, -11.5) -> (6.2, -16.5) projected
  line L90 (6.2, -16.5) -> (-6.2, -16.5) projected
  line L91 (-6.2, -16.5) -> (-6.2, -11.5) projected
  line L92 (-6.2, -11.5) -> (-6.2, 11.5) projected
  line L93 (-6.2, 11.5) -> (-6.2, 17.5) projected
  line L94 (-6.2, 17.5) -> (-4.5, 17.5) projected
  line L95 (81.8724, -71.3001) -> (94.3529, -115.1101) projected
  line L96 (-76.3482, -71.3001) -> (81.8724, -71.3001)
  arc A6 (-13.202, -156.6002) -> (13.202, -156.6002) centre (0, -156.6002) ccw projected
  line L97 (0, -169.8022) -> (0, 27.202)
  line L98 (-44.1, -88.4001) -> (44.1, -88.4001)
  line L99 (44.1, -88.4001) -> (44.1, -54.2001)
  line L100 (44.1, -54.2001) -> (-44.1, -54.2001)
  line L101 (-44.1, -54.2001) -> (-44.1, -88.4001)
  arc A7 (44.1, -88.4001) -> (44.1, -78.4001) centre (44.1, -83.4001) ccw
  arc A8 (44.1, -64.2001) -> (44.1, -54.2001) centre (44.1, -59.2001) ccw
  point P0 (0, 0)
  dimension "d523" = 88.2
  dimension "d524" = 34.2
  dimension "d525" = 17.1
  dimension "d526" = 44.1
  dimension "d527" = 5
  dimension "d528" = 5
  constraints: 12 end point, 7 point on circle, 2 centre point, 2 horizontal, 2 line through centre, 2 parallel, 2 point on line, 2 tangent, 1 perpendicular
  measures "d523" distance of L98.start L98.end
  measures "d524" distance of L98.end L99.end
  measures "d525" distance between parallel lines of L96 L98
  measures "d526" distance between parallel lines of L97 L99
  measures "d527" radius of A8
  measures "d528" radius of A7
extrude "Extrusion34" cut sketch "Sketch35" against normal blind 10 contours L98 L101 L96 L97 | L97 L96 L99 L98 | L97 L100 L99 L96 | L96 L101 L100 L97 | L99 A7 | L99 A8
sketch "Sketch36" plane through (0, 0, 10) normal (0, 0, 1) x (1, 0, 0)
  arc A0 (44.1, -64.2001) -> (44.1, -54.2001) centre (44.1, -59.2001) ccw projected
  line L0 (-44.1, -54.2001) -> (44.1, -54.2001) projected
  line L1 (-44.1, -88.4001) -> (-44.1, -54.2001) projected
  line L2 (44.1, -88.4001) -> (-44.1, -88.4001) projected
  arc A1 (44.1, -88.4001) -> (44.1, -78.4001) centre (44.1, -83.4001) ccw projected
  line L3 (44.1, -64.2001) -> (44.1, -78.4001) projected
  line L4 (-27.45, -57.3501) -> (29.15, -57.3501)
  line L5 (29.15, -57.3501) -> (29.15, -85.2501)
  line L6 (29.15, -85.2501) -> (-27.45, -85.2501)
  line L7 (-27.45, -85.2501) -> (-27.45, -57.3501)
  line L8 (-44.1, -54.2001) -> (44.1, -54.2001) projected
  line L9 (0, -54.2001) -> (0, -88.4001)
  line L10 (44.1, -88.4001) -> (-44.1, -88.4001) projected
  line L11 (44.1, -64.2001) -> (44.1, -78.4001) projected
  line L12 (44.1, -71.3001) -> (-44.1, -71.3001)
  line L13 (-44.1, -88.4001) -> (-44.1, -54.2001) projected
  line L14 (30.1, -62.4001) -> (24.1, -62.4001)
  line L15 (24.1, -62.4001) -> (24.1, -56.4001)
  line L16 (24.1, -56.4001) -> (30.1, -56.4001)
  line L17 (30.1, -56.4001) -> (30.1, -62.4001)
  line L18 (30.1, -62.4001) -> (24.1, -56.4001) construction
  line L19 (24.1, -62.4001) -> (30.1, -56.4001) construction
  line L20 (30.1, -80.2001) -> (24.1, -80.2001)
  line L21 (24.1, -80.2001) -> (24.1, -86.2001)
  line L22 (24.1, -86.2001) -> (30.1, -86.2001)
  line L23 (30.1, -86.2001) -> (30.1, -80.2001)
  line L24 (-30.1, -62.4001) -> (-24.1, -62.4001)
  line L25 (-24.1, -62.4001) -> (-24.1, -56.4001)
  line L26 (-24.1, -56.4001) -> (-30.1, -56.4001)
  line L27 (-30.1, -56.4001) -> (-30.1, -62.4001)
  line L28 (-30.1, -80.2001) -> (-24.1, -80.2001)
  line L29 (-24.1, -80.2001) -> (-24.1, -86.2001)
  line L30 (-30.1, -86.2001) -> (-30.1, -80.2001)
  line L31 (-24.1, -86.2001) -> (-30.1, -86.2001)
  line L32 (24.1, -46.4001) -> (30.1, -46.4001)
  line L33 (30.1, -46.4001) -> (30.1, -52.4001)
  line L34 (30.1, -52.4001) -> (24.1, -52.4001)
  line L35 (24.1, -52.4001) -> (24.1, -46.4001)
  line L36 (24.1, -46.4001) -> (30.1, -52.4001) construction
  line L37 (30.1, -46.4001) -> (24.1, -52.4001) construction
  line L38 (24.1, -96.2001) -> (30.1, -96.2001)
  line L39 (30.1, -96.2001) -> (30.1, -90.2001)
  line L40 (30.1, -90.2001) -> (24.1, -90.2001)
  line L41 (24.1, -90.2001) -> (24.1, -96.2001)
  line L42 (-24.1, -46.4001) -> (-30.1, -46.4001)
  line L43 (-30.1, -46.4001) -> (-30.1, -52.4001)
  line L44 (-30.1, -52.4001) -> (-24.1, -52.4001)
  line L45 (-24.1, -52.4001) -> (-24.1, -46.4001)
  line L46 (-30.1, -90.2001) -> (-24.1, -90.2001)
  line L47 (-24.1, -90.2001) -> (-24.1, -96.2001)
  line L48 (-24.1, -96.2001) -> (-30.1, -96.2001)
  line L49 (-30.1, -96.2001) -> (-30.1, -90.2001)
  point P0 (0, 0)
  point P1 (27.1, -59.4001)
  point P2 (27.1, -49.4001)
  point P3 (27.1, -49.4001)
  point P4 (27.1, -59.4001)
  dimension "d532" = 27.9
  dimension "d533" = 13.95
  dimension "d534" = 27.45
  dimension "d535" = 2.05
  dimension "d536" = 2.05
  dimension "d537" = 6
  dimension "d538" = 6
  dimension "d539" = 6
  dimension "d540" = 6
  dimension "d541" = 10
  dimension "d553" = 48.2
  constraints: 84 end point, 24 symmetric about line, 10 midpoint, 6 parallel, 3 horizontal, 3 perpendicular, 1 vertical alignment
  measures "d532" distance of L6.end L4.start
  measures "d533" distance between parallel lines of L12 L4
  measures "d534" distance between parallel lines of L9 L7
  measures "d535" distance from line of L5 point (27.1, -59.4)
  measures "d536" distance from line of L4 point (27.1, -59.4)
  measures "d537" distance of L14.end L15.end
  measures "d538" distance of L15.end L16.end
  measures "d539" distance of L33.end L34.end
  measures "d540" distance of L34.end L32.start
  measures "d541" distance of point (27.1, -49.4) point (27.1, -59.4)
  measures "d553" distance between parallel lines of L45 L35
extrude "Extrusion35" add sketch "Sketch36" along normal blind 25 contours L32 L33 L34 L35 | L41 L40 L39 L38 | L45 L44 L43 L42 | L46 L47 L48 L49
sketch "Sketch37" plane through (0, 0, 35) normal (0, 0, 1) x (1, 0, 0)
  line L0 (24.1, -96.2001) -> (30.1, -96.2001) projected
  line L1 (30.1, -96.2001) -> (30.1, -90.2001) projected
  line L2 (30.1, -90.2001) -> (24.1, -90.2001) projected
  line L3 (24.1, -90.2001) -> (24.1, -96.2001) projected
  line L4 (24.1, -52.4001) -> (30.1, -52.4001) projected
  line L5 (30.1, -52.4001) -> (30.1, -46.4001) projected
  line L6 (30.1, -46.4001) -> (24.1, -46.4001) projected
  line L7 (24.1, -46.4001) -> (24.1, -52.4001) projected
  line L8 (-30.1, -52.4001) -> (-24.1, -52.4001) projected
  line L9 (-24.1, -52.4001) -> (-24.1, -46.4001) projected
  line L10 (-24.1, -46.4001) -> (-30.1, -46.4001) projected
  line L11 (-30.1, -46.4001) -> (-30.1, -52.4001) projected
  line L12 (-24.1, -96.2001) -> (-24.1, -90.2001) projected
  line L13 (-24.1, -90.2001) -> (-30.1, -90.2001) projected
  line L14 (-30.1, -90.2001) -> (-30.1, -96.2001) projected
  line L15 (-30.1, -96.2001) -> (-24.1, -96.2001) projected
  line L16 (30.1, -90.2001) -> (24.1, -90.2001)
  line L17 (24.1, -90.2001) -> (24.1, -71.3001)
  line L18 (24.1, -71.3001) -> (30.1, -71.3001)
  line L19 (30.1, -71.3001) -> (30.1, -90.2001)
  line L20 (30.1, -52.4001) -> (24.1, -52.4001)
  line L21 (24.1, -52.4001) -> (24.1, -71.3001)
  line L22 (24.1, -71.3001) -> (30.1, -71.3001)
  line L23 (30.1, -71.3001) -> (30.1, -52.4001)
  line L24 (-24.1, -90.2001) -> (-30.1, -90.2001)
  line L25 (-30.1, -90.2001) -> (-30.1, -71.3001)
  line L26 (-30.1, -71.3001) -> (-24.1, -71.3001)
  line L27 (-24.1, -71.3001) -> (-24.1, -90.2001)
  line L28 (-30.1, -52.4001) -> (-24.1, -52.4001) projected
  line L29 (-24.1, -52.4001) -> (-30.1, -52.4001)
  line L30 (-30.1, -52.4001) -> (-30.1, -71.3001)
  line L31 (-30.1, -71.3001) -> (-24.1, -71.3001)
  line L32 (-24.1, -71.3001) -> (-24.1, -52.4001)
  line L33 (-24.1, -71.3001) -> (-24.1, -59.4001)
  circle A0 centre (-25.4, -59.4001) radius 1.25
  line L34 (-24.1, -71.3001) -> (24.1, -71.3001)
  line L35 (-6.2, -16.5) -> (6.2, -16.5) projected
  line L36 (0, -16.5) -> (0, -126.1002)
  line L37 (-6.2, -126.1002) -> (6.2, -126.1002) projected
  circle A1 centre (25.4, -59.4001) radius 1.25
  circle A2 centre (-25.4, -83.2001) radius 1.25
  circle A3 centre (25.4, -83.2001) radius 1.25
  point P0 (0, 0)
  dimension "d544" = 18.9
  dimension "d545" = 6
  dimension "d546" = 18.9
  dimension "d547" = 6
  dimension "d548" = 18.9
  dimension "d549" = 6
  dimension "d550" = 18.9
  dimension "d554" = 11.9
  dimension "d555" = 2.5
  dimension "d556" = 1.3
  dimension "d557" = 23.8
  constraints: 38 end point, 8 parallel, 4 centre point, 4 horizontal, 4 perpendicular, 3 symmetric about line, 2 midpoint, 2 point on line, 3 other
  measures "d544" distance of L16.end L17.end
  measures "d545" distance of L17.end L18.end
  measures "d546" distance of L20.end L21.end
  measures "d547" distance of L21.end L22.end
  measures "d548" distance of L24.end L25.end
  measures "d549" distance of L25.end L26.end
  measures "d550" distance of L29.end L30.end
  measures "d554" distance of L31.end L33.end
  measures "d555" diameter of A0
  measures "d556" distance of L33.end A0.centre
  measures "d557" distance of A2.centre A0.centre
extrude "Extrusion36" add sketch "Sketch37" against normal blind 10 contours L17 L18 L19 L2 | L21 L4 L23 L18 | L8 L32 L26 L30 | L26 L27 L13 L25 | A0 | A1 | A2 | A3
extrude "Extrusion37" cut sketch "Sketch37" against normal blind 20 contours A0 | A1 | A2 | A3
sketch "Sketch38" plane through (0, 0, 25) normal (0, 0, -1) x (-1, 0, 0)
  circle A0 centre (25.4, -59.4001) radius 0.865
  circle A1 centre (25.4, -83.2001) radius 0.865
  circle A2 centre (-25.4, -83.2001) radius 0.865
  circle A3 centre (-25.4, -59.4001) radius 0.865
  line L0 (-27.1898, -56.3001) -> (-23.6102, -56.3001)
  line L1 (-23.6102, -56.3001) -> (-21.8204, -59.4001)
  line L2 (-21.8204, -59.4001) -> (-23.6102, -62.5001)
  line L3 (-23.6102, -62.5001) -> (-27.1898, -62.5001)
  line L4 (-27.1898, -62.5001) -> (-28.9796, -59.4001)
  line L5 (-28.9796, -59.4001) -> (-27.1898, -56.3001)
  circle A4 centre (-25.4, -83.2001) radius 1.25 projected
  line L6 (-27.1898, -80.1001) -> (-23.6102, -80.1001)
  line L7 (-23.6102, -80.1001) -> (-21.8204, -83.2001)
  line L8 (-21.8204, -83.2001) -> (-23.6102, -86.3001)
  line L9 (-23.6102, -86.3001) -> (-27.1898, -86.3001)
  line L10 (-27.1898, -86.3001) -> (-28.9796, -83.2001)
  line L11 (-28.9796, -83.2001) -> (-27.1898, -80.1001)
  line L12 (27.1898, -56.3001) -> (28.9796, -59.4001)
  line L13 (28.9796, -59.4001) -> (27.1898, -62.5001)
  line L14 (27.1898, -62.5001) -> (23.6102, -62.5001)
  line L15 (23.6102, -62.5001) -> (21.8204, -59.4001)
  line L16 (21.8204, -59.4001) -> (23.6102, -56.3001)
  line L17 (23.6102, -56.3001) -> (27.1898, -56.3001)
  circle A5 centre (25.4, -83.2001) radius 1.25 projected
  line L18 (27.1898, -80.1001) -> (28.9796, -83.2001)
  line L19 (28.9796, -83.2001) -> (27.1898, -86.3001)
  line L20 (27.1898, -86.3001) -> (23.6102, -86.3001)
  line L21 (23.6102, -86.3001) -> (21.8204, -83.2001)
  line L22 (21.8204, -83.2001) -> (23.6102, -80.1001)
  line L23 (23.6102, -80.1001) -> (27.1898, -80.1001)
  line L24 (-30.1, -46.4001) -> (-24.1, -46.4001) projected
  line L25 (24.1, -46.4001) -> (30.1, -46.4001) projected
  point P0 (0, 0)
  dimension "d560" = 3.1
  dimension "d561" = 3.1
  dimension "d562" = 3.1
  dimension "d563" = 3.1
  constraints: 48 end point, 4 centre point, 4 coincident, 4 parallel, 60 other
  measures "d560" distance from line of L0 A3.centre
  measures "d561" distance from line of L6 A2.centre
  measures "d562" distance from line of L23 A1.centre
  measures "d563" distance from line of L17 A0.centre
extrude "Extrusion38" cut sketch "Sketch38" against normal blind 2.4 contours A0 | A1 | A2 | A3 | L0 L1 L2 L3 L4 L5 | A4 | L6 L7 L8 L9 L10 L11 | L12 L13 L14 L15 L16 L17 | A5 | L18 L19 L20 L21 L22 L23